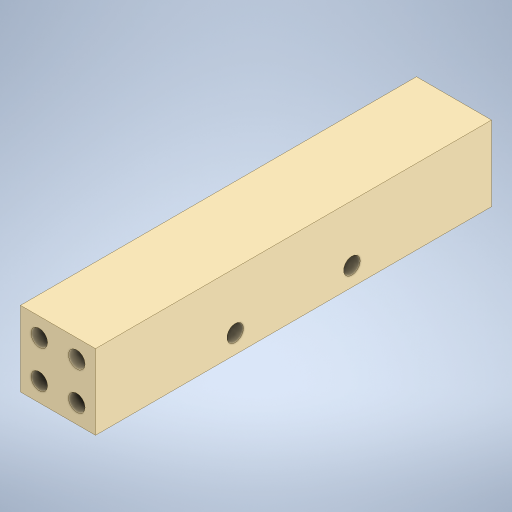
# Autodesk Inventor part: HUDSON 1-02-REAR DRAWBAR BEAM
Saved by Autodesk Inventor 2024.2 (Build 282272000, 272)
## iProperties
Created: 2024-09-29
Part Number: HUDSON 1-02-REAR DRAWBAR BEAM
Material: Generic
Document SubType Name: Modeling
Designer: Jimena Brenes
Density: 1 g/cm^3
Appearance: Beige
Author: Jimena Brenes
Autodesk Inventor part; units mm, degrees
ref_plane "YZ Plane" through (0, 0, 0) normal (1, 0, 0) x (0, 1, 0)
ref_plane "XZ Plane" through (0, 0, 0) normal (0, 1, 0) x (-1, 0, 0)
ref_plane "XY Plane" through (0, 0, 0) normal (0, 0, 1) x (1, 0, 0)
sketch "Sketch1" plane through (0, 0, 0) normal (0, 0, 1) x (1, 0, 0)
  line L0 (0, 0) -> (18, 0)
  line L1 (18, 0) -> (18, 18)
  line L2 (18, 18) -> (0, 18)
  line L3 (0, 18) -> (0, 0)
  line L4 (13.5, 4.5) -> (4.5, 4.5) construction
  line L5 (4.5, 4.5) -> (4.5, 13.5) construction
  line L6 (4.5, 13.5) -> (13.5, 13.5) construction
  line L7 (13.5, 13.5) -> (13.5, 4.5) construction
  line L8 (13.5, 4.5) -> (4.5, 13.5) construction
  line L9 (4.5, 4.5) -> (13.5, 13.5) construction
  circle A0 centre (4.5, 13.5) radius 2
  circle A1 centre (13.5, 13.5) radius 2
  circle A2 centre (4.5, 4.5) radius 2
  circle A3 centre (13.5, 4.5) radius 2
  point P0 (9, 9)
  dimension "d0" = 18
  dimension "d1" = 18
  dimension "d2" = 4
  dimension "d3" = 4
  dimension "d5" = 4
  dimension "d6" = 4
  dimension "d7" = 4.5
  dimension "d8" = 9
  dimension "d9" = 9
  dimension "d10" = 4.5
  constraints: 20 end point, 4 centre point, 4 coincident, 4 parallel, 2 horizontal, 2 midpoint, 2 perpendicular
  measures "d0" distance between parallel lines of L1 L3
  measures "d1" distance between parallel lines of L0 L2
  measures "d2" diameter of A0
  measures "d3" diameter of A1
  measures "d5" diameter of A2
  measures "d6" diameter of A3
  measures "d7" distance from line of L3 A2.centre
  measures "d8" distance of L4.end L4.start
  measures "d9" distance of L4.start L6.end
  measures "d10" distance from line of L2 L6.end
extrude "Extrusion1" add sketch "Sketch1" against normal blind 95 contours L3 L2 L1 L0 | A0 | A1 | A2 | A3
hole "Hole1" at (4.5, 13.5, 0) at (4.5, 4.5, 0) at (13.5, 13.5, 0) at (13.5, 4.5, 0) direction (0, 0, -1) diameter 4 depth 10 tip angle 118
sketch "Sketch2" plane through (18, 0, 0) normal (1, 0, 0) x (0, 0, -1)
  circle A0 centre (33.5, 4.5) radius 2
  circle A1 centre (61.5, 4.5) radius 2
  line L0 (0, 0) -> (0, 18) projected
  line L1 (95, 18) -> (95, 0) projected
  line L2 (0, 0) -> (95, 0) projected
  dimension "d20" = 4
  dimension "d21" = 4
  dimension "d22" = 33.5
  dimension "d23" = 28
  dimension "d24" = 33.5
  dimension "d25" = 4.5
  constraints: 2 centre point
  measures "d20" diameter of A0
  measures "d21" diameter of A1
  measures "d22" distance from line of L0 A0.centre
  measures "d23" distance of A1.centre A0.centre
  measures "d24" distance from line of L1 A1.centre
  measures "d25" distance from line of L2 A1.centre
hole "Hole2" at (18, 4.5, -33.5) at (18, 4.5, -61.5) direction (-1, 0, 0) diameter 4 depth 10 tip angle 118
sketch "Sketch3" plane through (0, 0, 0) normal (0, -1, 0) x (1, 0, 0)
  circle A0 centre (6, -11) radius 1.5
  circle A1 centre (6, -20) radius 1.5
  circle A2 centre (6, -65.5) radius 1.5
  circle A3 centre (6, -88.5) radius 1.5
  line L0 (0, 0) -> (18, 0) projected
  line L1 (0, 0) -> (0, -95) projected
  dimension "d33" = 3
  dimension "d34" = 3
  dimension "d35" = 3
  dimension "d36" = 3
  dimension "d37" = 11
  dimension "d38" = 9
  dimension "d39" = 6
  dimension "d40" = 6
  dimension "d41" = 45.5
  dimension "d42" = 6
  dimension "d43" = 23
  dimension "d44" = 6
  constraints: 4 centre point
  measures "d33" diameter of A0
  measures "d34" diameter of A1
  measures "d35" diameter of A2
  measures "d36" diameter of A3
  measures "d37" distance from line of L0 A0.centre
  measures "d38" distance of A1.centre A0.centre
  measures "d39" distance from line of L1 A0.centre
  measures "d40" distance from line of L1 A1.centre
  measures "d41" distance of A1.centre A2.centre
  measures "d42" distance from line of L1 A2.centre
  measures "d43" distance of A3.centre A2.centre
  measures "d44" distance from line of L1 A3.centre
hole "Hole3" at (6, 0, -11) at (6, 0, -20) at (6, 0, -65.5) at (6, 0, -88.5) direction (0, 1, 0) diameter 3 depth 10 tip angle 118
sketch "Sketch4" plane through (0, 0, -95) normal (0, 0, -1) x (-1, 0, 0)
  line L0 (-4.5, 4.5) -> (-13.5, 4.5) construction
  line L1 (-13.5, 4.5) -> (-13.5, 13.5) construction
  line L2 (-13.5, 13.5) -> (-4.5, 13.5) construction
  line L3 (-4.5, 13.5) -> (-4.5, 4.5) construction
  line L4 (-4.5, 4.5) -> (-13.5, 13.5) construction
  line L5 (-13.5, 4.5) -> (-4.5, 13.5) construction
  circle A0 centre (-4.5, 13.5) radius 2
  circle A1 centre (-13.5, 13.5) radius 2
  circle A2 centre (-4.5, 4.5) radius 2
  line L6 (-18, 18) -> (-18, 0) projected
  line L7 (0, 18) -> (-18, 18) projected
  line L8 (-18, 0) -> (0, 0) projected
  circle A3 centre (-13.5, 4.5) radius 2
  point P0 (-9, 9)
  dimension "d52" = 4
  dimension "d53" = 4
  dimension "d55" = 4
  dimension "d56" = 9
  dimension "d57" = 4.5
  dimension "d58" = 4.5
  dimension "d59" = 9
  dimension "d61" = 4.5
  dimension "d62" = 9
  dimension "d63" = 4
  constraints: 12 end point, 4 centre point, 4 coincident, 2 midpoint, 2 parallel, 1 horizontal, 1 perpendicular
  measures "d52" diameter of A0
  measures "d53" diameter of A1
  measures "d55" diameter of A2
  measures "d56" distance of L0.end L1.end
  measures "d57" distance from line of L6 L0.end
  measures "d58" distance from line of L7 L1.end
  measures "d59" distance of L1.end L2.end
  measures "d61" distance from line of L8 L0.start
  measures "d62" distance of L0.start L2.end
  measures "d63" diameter of A3
hole "Hole4" at (13.5, 13.5, -95) at (13.5, 4.5, -95) at (4.5, 13.5, -95) at (4.5, 4.5, -95) direction (0, 0, 1) diameter 4 depth 10 tip angle 118
body "Solid1"
